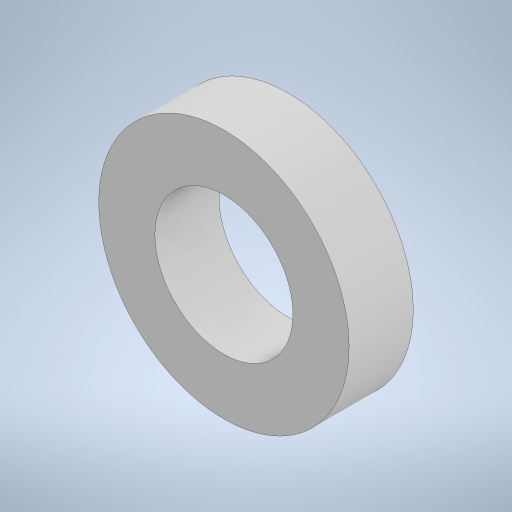
# Autodesk Inventor part: TulejaKołoV2
Saved by Autodesk Inventor 2024 (Build 280153000, 153)
## iProperties
Created: 2025-03-19
Part Number: TulejaKołoV2
Material: Ogólny
Document SubType Name: Modeling
Designer: Victoria
Density: 1 g/cm^3
Appearance: Domyślna
Author: Victoria
Autodesk Inventor part; units mm, degrees
ref_plane "YZ Plane" through (0, 0, 0) normal (1, 0, 0) x (0, 1, 0)
ref_plane "XZ Plane" through (0, 0, 0) normal (0, 1, 0) x (-1, 0, 0)
ref_plane "XY Plane" through (0, 0, 0) normal (0, 0, 1) x (1, 0, 0)
sketch "Szkic1" plane through (0, 0, 0) normal (0, 0, 1) x (1, 0, 0)
  circle A0 centre (0, 0) radius 2.15
  circle A1 centre (0, 0) radius 3.9
  dimension "d0" = 4.3
  dimension "d4" = 7.8
  constraints: 2 centre point, 2 coincident
  measures "d0" diameter of A0
  measures "d4" diameter of A1
extrude "Wyciągnięcie proste1" add sketch "Szkic1" along normal blind 2
